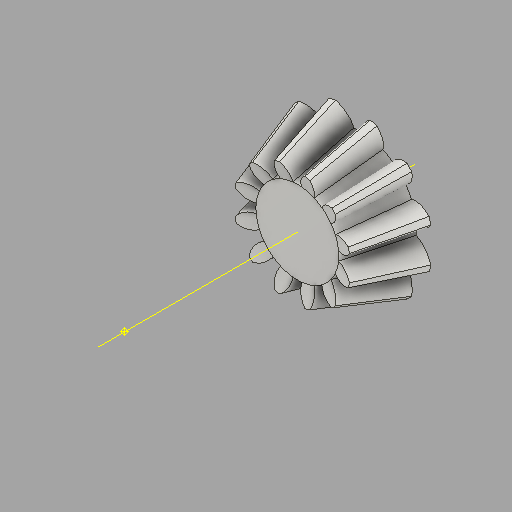
# Autodesk Inventor part: Bevel Gear1
Saved by Autodesk Inventor 2024 (Build 280153000, 153)
## iProperties
Created: 2024-04-12
Part Number: Bevel Gear1
Material: Steel, Mild
Document SubType Name: Modeling
Designer: Alex
Categories: <?xml version="1.0" encoding="UTF-16"?> <MemberInstance><Categories><FamilyTemplate><FamilyTemplateParameter ValueType="xs:double" Id="1" ObjectReferenceKey="da_z" ObjectType="kUserParameterObject"/><FamilyTemplateParameter ValueType="xs:double" Id="2" ObjectReferenceKey="da_b" ObjectType="kUserParameterObject"/><FamilyTemplateParameter ValueType="xs:double" Id="3" ObjectReferenceKey="da_beta" ObjectType="kUserParameterObject"/><FamilyTemplateParameter ValueType="xs:double" Id="4" ObjectReferenceKey="da_dae" ObjectType="kUserParameterObject"/><FamilyTemplateParameter ValueType="xs:double" Id="5" ObjectReferenceKey="da_ve" ObjectType="kUserParameterObject"/><FamilyTemplateParameter ValueType="xs:double" Id="6" ObjectReferenceKey="da_omega" ObjectType="kUserParameterObject"/><FamilyTemplateParameter ValueType="xs:string" Id="7" ObjectReferenceKey="EAIAABAAAAAAHwAAAAAAAIAAAAAAAAAA" ObjectType="83914240" SubObjectId="SurfaceGeometry"/></FamilyTemplate><ParamToTemplateMap><ParamToTemplate CategoryParameter="//CategoryParameter[@InternalName='046C89C9-8512-4d59-83FE-43B91F4F132A']" TemplateParameter="1"/><ParamToTemplate CategoryParameter="//CategoryParameter[@InternalName='2552DF32-E462-4b46-AEBF-C6C7768E72AC']" TemplateParameter="2"/><ParamToTemplate CategoryParameter="//CategoryParameter[@InternalName='C9EE641D-15FC-4fae-A226-E94C4372FDD7']" TemplateParameter="3"/><ParamToTemplate><ParamToTemplate CategoryParameter="//CategoryParameter[@InternalName='00B6519A-459B-49c7-AD84-2E56D39A5744']" ConstantValue="0.000000"/></ParamToTemplate><ParamToTemplate><ParamToTemplate CategoryParameter="//CategoryParameter[@InternalName='04B31F0E-C7A6-4894-AA32-9629BEFACF47']" ConstantValue="1.000000"/></ParamToTemplate><ParamToTemplate><ParamToTemplate CategoryParameter="//CategoryParameter[@InternalName='43CBEC2E-7847-49e7-A936-2F7889FCB2D9']" ConstantValue="0.200000"/></ParamToTemplate><ParamToTemplate><ParamToTemplate CategoryParameter="//CategoryParameter[@InternalName='B1EFC894-105D-4ebd-86BF-FA20ED196853']" ConstantValue="0.269800"/></ParamToTemplate><ParamToTemplate><ParamToTemplate CategoryParameter="//CategoryParameter[@InternalName='51175063-3D10-4879-93E8-6246FE8B403D']" ConstantValue="2060000000.000000"/></ParamToTemplate><ParamToTemplate><ParamToTemplate CategoryParameter="//CategoryParameter[@InternalName='A3A52E27-4454-46a9-B0BD-C932399B70AF']" ConstantValue="0.300000"/></ParamToTemplate><ParamToTemplate CategoryParameter="//CategoryParameter[@InternalName='2A200944-5A8C-41ca-B96E-8520D2E510F1']" TemplateParameter="4"/><ParamToTemplate><ParamToTemplate CategoryParameter="//CategoryParameter[@InternalName='1A637F62-92C8-44bc-B81F-10802510B579']" ConstantValue="1.515315"/></ParamToTemplate><ParamToTemplate CategoryParameter="//CategoryParameter[@InternalName='B52DD4BE-6863-48fb-BF58-89EF6F9EC65C']" TemplateParameter="5"/><ParamToTemplate><ParamToTemplate CategoryParameter="//CategoryParameter[@InternalName='3956BFF2-84D2-457d-93C2-9B0613DEBA67']" ConstantValue="2.176157"/></ParamToTemplate><ParamToTemplate CategoryParameter="//CategoryParameter[@InternalName='739CFA02-461B-4bf8-8049-181FCAD8B28F']" TemplateParameter="6"/><ParamToTemplate><ParamToTemplate CategoryParameter="//CategoryParameter[@InternalName='A27E999F-E2CE-4481-8A2A-EBF499C4C3C5']" ConstantValue="0.000000"/></ParamToTemplate><ParamToTemplate><ParamToTemplate CategoryParameter="//CategoryParameter[@InternalName='9E1B4470-B2D3-4ff1-B813-535BB4CDF51A']" ConstantValue="5000000.000000"/></ParamToTemplate><ParamToTemplate><ParamToTemplate CategoryParameter="//CategoryParameter[@InternalName='F8452263-BFF6-458c-9FB1-07C4B99E95CD']" ConstantValue="11400000.000000"/></ParamToTemplate><ParamToTemplate><ParamToTemplate CategoryParameter="//CategoryParameter[@InternalName='3E3BB259-FD49-497f-8171-6EBC954A3479']" ConstantValue="2.000000"/></ParamToTemplate><ParamToTemplate CategoryParameter="//CategoryParameter[@InternalName='27C3BAF2-7550-4e4b-AE2C-0DB134B7D9B7']" TemplateParameter="7"/></ParamToTemplateMap><Category DisplayName="Gear" InternalName="DC85795E-93AB-48d5-8EEE-5A27447B64BD" Mnemonic="Gear"><CategoryParameter DisplayName="z" InternalName="046C89C9-8512-4d59-83FE-43B91F4F132A" Mnemonic="z"/><CategoryParameter DisplayName="b" InternalName="2552DF32-E462-4b46-AEBF-C6C7768E72AC" Mnemonic="b"/><CategoryParameter DisplayName="||b|" InternalName="C9EE641D-15FC-4fae-A226-E94C4372FDD7" Mnemonic="beta"/><CategoryParameter DisplayName="x" InternalName="00B6519A-459B-49c7-AD84-2E56D39A5744" Mnemonic="x"/><CategoryParameter DisplayName="a*" InternalName="04B31F0E-C7A6-4894-AA32-9629BEFACF47" Mnemonic="a"/><CategoryParameter DisplayName="c*" InternalName="43CBEC2E-7847-49e7-A936-2F7889FCB2D9" Mnemonic="c"/><CategoryParameter DisplayName="r|.f|*" InternalName="B1EFC894-105D-4ebd-86BF-FA20ED196853" Mnemonic="rf"/><CategoryParameter DisplayName="E" InternalName="51175063-3D10-4879-93E8-6246FE8B403D" Mnemonic="E"/><CategoryParameter DisplayName="||m|" InternalName="A3A52E27-4454-46a9-B0BD-C932399B70AF" Mnemonic="mi"/><Category DisplayName="BevelGear" InternalName="0C98F69A-0C2B-4791-B2FE-7691BB227E77" Mnemonic="BevelGear"><CategoryParameter DisplayName="d|.ae|" InternalName="2A200944-5A8C-41ca-B96E-8520D2E510F1" Mnemonic="dae"/><CategoryParameter DisplayName="d|.ai|" InternalName="1A637F62-92C8-44bc-B81F-10802510B579" Mnemonic="dai"/><CategoryParameter DisplayName="A|.e|" InternalName="B52DD4BE-6863-48fb-BF58-89EF6F9EC65C" Mnemonic="ve"/><CategoryParameter DisplayName="A|.i|" InternalName="3956BFF2-84D2-457d-93C2-9B0613DEBA67" Mnemonic="vi"/><CategoryParameter DisplayName="||S|" InternalName="739CFA02-461B-4bf8-8049-181FCAD8B28F" Mnemonic="omega"/><CategoryParameter DisplayName="x|.t|" InternalName="A27E999F-E2CE-4481-8A2A-EBF499C4C3C5" Mnemonic="xt"/><CategoryParameter DisplayName="||s||.Flim|" InternalName="9E1B4470-B2D3-4ff1-B813-535BB4CDF51A" Mnemonic="sFlim"/><CategoryParameter DisplayName="||s||.Hlim|" InternalName="F8452263-BFF6-458c-9FB1-07C4B99E95CD" Mnemonic="sHlim"/><CategoryParameter DisplayName="type" InternalName="3E3BB259-FD49-497f-8171-6EBC954A3479" Mnemonic="type"/><CategoryParameter DisplayName="PitchDiameter" InternalName="27C3BAF2-7550-4e4b-AE2C-0DB134B7D9B7" Mnemonic="IDS_PITCHDIAM"/></Category></Category></Categories></MemberInstance>
Mass: 60.9118 g
Surface Area: 34.3074 cm^2
Volume: 7.7496 cm^3
Density: 7.86 g/cm^3
Appearance: Steel
CustomPartVersion: 1
Author: Alex
Autodesk Inventor part; units mm, degrees
ref_plane "Mesh Plane2" through (0, 0, 0) normal (0.9659258, 0.258819, 0) x (0, 0, 1)
sketch "Teeth Body Sketch" plane through (0, 0, 0) normal (1, 0, 0) x (0, 1, 0)
  line L0 (0, 0) -> (7.2759, -30.5172) construction
  line L1 (7.2759, -30.5172) -> (10.3082, -29.6075)
  line L2 (10.3082, -29.6075) -> (0, 0) construction
  line L3 (9, -30) -> (0, 0) construction
  line L4 (5.3478, -22.4302) -> (7.5766, -21.7616)
  line L5 (7.2759, -30.5172) -> (5.3478, -22.4302)
  line L6 (10.3082, -29.6075) -> (7.5766, -21.7616)
  line L7 (0, -39.3868) -> (0, 6.5645) projected
  line L8 (0, -30) -> (10.3082, -30) construction
  dimension "d0" = 18
  dimension "d1" = 14.5518
  dimension "d2" = 20.6165
  dimension "d3" = 8.3
  dimension "d4" = 29.6075
  constraints: 16 end point, 4 point on line, 3 perpendicular, 2 collinear, 1 horizontal alignment, 1 vertical alignment
  measures "d0" diameter of L3.start L7
  measures "d1" diameter of L0.end L7
  measures "d2" diameter of L1.end L7
  measures "d3" distance between parallel lines of L1 L4
  measures "d4" vertical distance of L1.end L0.start
revolve "Teeth Body" add sketch "Teeth Body Sketch" angle 360 about axis through (0, 0, 0) along (0, 0, 1)
ref_plane "Tooth Plane" through (0, 9, -30) normal (0, -0.2873479, 0.9578263) x (1, 0, 0)
sketch "Start Sketch" plane through (0, 9, -30) normal (0, -0.2873479, 0.9578263) x (1, 0, 0)
  line L0 (0, -23.5051) -> (0, 10.6448) projected
  arc A0 (-0.8153, -2.1799) -> (-3.6557, 1.7305) centre (-4.2772, -1.7078) ccw
  arc A1 (3.6557, 1.7305) -> (0.8153, -2.1799) centre (4.2772, -1.7078) ccw
  line L1 (-0.8153, -2.1799) -> (0.8153, -2.1799)
  arc A2 (3.6557, 1.7305) -> (-3.6557, 1.7305) centre (0, -9.3963) ccw
  dimension "d7" = 3.494
  dimension "d8" = 4.2772
  dimension "d9" = 7.6885
  dimension "d57" = 11.7119
  dimension "d58" = 7.2164
  constraints: 6 point on circle, 3 centre point, 3 symmetric about line, 2 end point, 1 coincident, 1 perpendicular, 1 other
  measures "d7" radius of A0
  measures "d8" horizontal distance of point (0, -9.396) A0.centre
  measures "d9" vertical distance of point (0, -9.396) A0.centre
  measures "d57" radius of A2
  measures "d58" distance from line of A2.centre L1
sketch "End Sketch" plane through (0, 6.5695, -21.8984) normal (0, -0.2873479, 0.9578263) x (1, 0, 0)
  line L0 (0, -15.354) -> (0, 6.9534) projected
  arc A0 (-0.5951, -1.5912) -> (-2.6685, 1.2631) centre (-3.1221, -1.2466) ccw
  arc A1 (2.6685, 1.2631) -> (0.5951, -1.5912) centre (3.1221, -1.2466) ccw
  line L1 (-0.5951, -1.5912) -> (0.5951, -1.5912)
  arc A2 (2.6685, 1.2631) -> (-2.6685, 1.2631) centre (0, -6.8588) ccw
  dimension "d12" = 2.5504
  dimension "d15" = 3.1221
  dimension "d16" = 5.6122
  dimension "d59" = 8.5491
  dimension "d60" = 5.2676
  constraints: 6 point on circle, 3 centre point, 3 symmetric about line, 2 end point, 1 coincident, 1 other
  measures "d12" radius of A0
  measures "d15" horizontal distance of A0.centre point (0, -6.859)
  measures "d16" vertical distance of A0.centre point (0, -6.859)
  measures "d59" radius of A2
  measures "d60" distance from line of A2.centre L1
loft "Loft" cut profiles "Start Sketch", "End Sketch"
pattern_circular "Circular Pattern" count 12 over 360 about axis through (0, 0, 0) along (0, 0, 1) of "Loft"
ref_plane "End Plane" through (0, 6.5695, -21.8984) normal (0, -0.2873479, 0.9578263) x (1, 0, 0)
sketch3d "3D Sketch Right"
ref_plane "End Plane Right" through (-2.5238, 6.0654, -21.8984) normal (0.1103904, -0.2652975, 0.9578263) x (0.9232624, 0.3841699, 0)
sketch "End Sketch Right" plane through (-2.5238, 6.0654, -21.8984) normal (0.1103904, -0.2652975, 0.9578263) x (0.9232624, 0.3841699, 0)
  arc A0 (-0.5951, -1.5912) -> (-2.6685, 1.2631) centre (-3.1221, -1.2466) ccw
  line L0 (0, -21.6214) -> (0, 13.2208) projected
  arc A1 (2.6685, 1.2631) -> (0.5951, -1.5912) centre (3.1221, -1.2466) ccw
  line L1 (-0.5951, -1.5912) -> (0.5951, -1.5912)
  arc A2 (2.6685, 1.2631) -> (-2.6685, 1.2631) centre (0, -6.8588) ccw
  dimension "d70" = 3.1221
  dimension "d71" = 5.6122
  dimension "d72" = 2.5504
  dimension "d73" = 5.2676
  dimension "d74" = 8.5491
  constraints: 6 point on circle, 3 centre point, 3 symmetric about line, 2 end point, 1 coincident, 1 perpendicular, 1 other
  measures "d70" horizontal distance of A2.centre A0.centre
  measures "d71" vertical distance of point (0, -6.859) A0.centre
  measures "d72" radius of A0
  measures "d73" distance from line of point (0, -6.859) L1
  measures "d74" radius of A2
feature "Loft Right" [suppressed]
pattern_circular "Circular Pattern Right" [suppressed]
sketch3d "3D Sketch Left"
ref_plane "End Plane Left" through (2.516, 6.0654, -21.896) normal (-0.1100652, -0.2653344, 0.9578535) x (0.9236824, -0.383159, 0)
sketch "End Sketch Left" plane through (2.516, 6.0654, -21.896) normal (-0.1100652, -0.2653344, 0.9578535) x (0.9236824, -0.383159, 0)
  line L0 (0, -38.185) -> (0, 21.1622) projected
  arc A0 (-0.5951, -1.589) -> (-2.6685, 1.2653) centre (-3.1221, -1.2444) ccw
  arc A1 (2.6685, 1.2653) -> (0.5951, -1.589) centre (3.1221, -1.2444) ccw
  line L1 (-0.5951, -1.589) -> (0.5951, -1.589)
  ellipse E0 centre (0, -6.2512) end of major axis (7.5766, -6.2512) minor radius 7.2573 projected
  arc A2 (2.6685, 1.2653) -> (-2.6685, 1.2653) centre (0, -6.8566) ccw
  dimension "d56" = 7.2572
  dimension "d30" = 2.5504
  dimension "d31" = 3.1221
  dimension "d32" = 5.6122
  dimension "d61" = 8.5491
  dimension "d62" = 5.2676
  constraints: 6 point on circle, 3 centre point, 3 symmetric about line, 2 end point, 1 coincident, 2 other
  measures "d30" radius of A0
  measures "d31" horizontal distance of point (0, -6.857) A0.centre
  measures "d32" vertical distance of A0.centre point (0, -6.857)
  measures "d61" radius of A2
  measures "d62" distance from line of point (0, -6.857) L1
feature "Loft Left" [suppressed]
pattern_circular "Circular Pattern Left" [suppressed]
sketch "Body Sketch" plane through (0, 0, 0) normal (1, 0, 0) x (0, 1, 0)
  line L0 (0, -35.0375) -> (0, -19.5308) projected
  line L1 (7.2759, -30.5172) -> (5.3478, -22.4302) projected
  line L2 (5.3478, -22.4302) -> (0, -22.4302)
  line L3 (7.2759, -30.5172) -> (0, -30.5172)
  constraints: 4 end point, 2 perpendicular, 2 point on line
revolve "Fix Body" add sketch "Body Sketch" angle 360 about axis through (0, 0, 0) along (0, 0, 1)
sketch "Sketch6" plane through (0, 0, 0) normal (1, 0, 0) x (0, 1, 0)
  line L0 (9, -30) -> (0, 0) projected
  line L1 (0, -37.7999) -> (0, 6.3) projected
surface revolve "Pitch Diameter" sketch "Sketch6" angle 360 about axis through (0, 0, 0) along (0, 0, 1) shown no curves L0
equation "\"d0\" = da_de"
equation "\"d1\" = da_dfe"
equation "\"d2\" = da_dae"
equation "\"d3\" = da_b"
equation "\"d4\" = da_ve"
equation "\"d7\" = fd_rr"
equation "\"d8\" = fd_x"
equation "\"d9\" = fd_y"
equation "\"d57\" = 0.5 * fd_dva + 0.3 * da_he"
equation "\"d58\" = 0.5 * fd_dva - 1.12 * da_he"
equation "\"da_teethtype\" = 0"
equation "\"da_b\" = 8.3"
equation "\"da_de\" = 18"
equation "\"da_dae\" = 20.6165"
equation "\"da_dfe\" = 14.55183"
equation "\"da_le\" = 31.32092"
equation "\"da_omega\" = 90deg"
equation "\"da_beta\" = 0"
equation "\"da_delta\" = 16.699244deg"
equation "\"da_alpha\" = 20deg"
equation "\"da_he\" = 3.16585"
equation "\"da_ve\" = 29.60753"
equation "\"da_zv\" = 12.528368"
equation "\"fd_loft\" = da_b + 0.05 * da_he"
equation "\"fd_x\" = fd_x1 + fd_x2"
equation "\"fd_y\" = fd_y1 - fd_y2"
equation "\"fd_dd\" = fd_dva - 0.8 * da_he"
equation "\"da_dvw\" = 18.79255"
equation "\"d11\" = fd_loft"
equation "\"da_dm\" = 15.61501"
equation "\"da_x\" = 0"
equation "\"da_m\" = 1.5"
equation "\"d50\" = da_omega"
equation "\"fd_rr\" = 3.493985"
equation "\"fd_dva\" = 21.524254"
equation "\"fd_x1\" = 1.187999"
equation "\"fd_x2\" = 3.089209"
equation "\"fd_y1\" = 9.320872"
equation "\"fd_y2\" = 1.632397"
body "Solid1"
body "Srf1"
